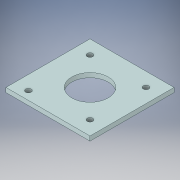
# Autodesk Inventor part: BASE_SOST.MEDIO
Saved by Autodesk Inventor 2019 (Build 230136000, 136)
## iProperties
Created: 2020-02-12
Part Number: BASE_SOST.MEDIO
Material: Genérico
Document SubType Name: Modeling
Designer: omar-
Density: 1 g/cm^3
Appearance: Valor por defecto
Author: omar-
Autodesk Inventor part; units mm, degrees
ref_plane "YZ Plane" through (0, 0, 0) normal (1, 0, 0) x (0, 1, 0)
ref_plane "XZ Plane" through (0, 0, 0) normal (0, 1, 0) x (-1, 0, 0)
ref_plane "XY Plane" through (0, 0, 0) normal (0, 0, 1) x (1, 0, 0)
sketch "Boceto1" plane through (0, 0, 0) normal (0, 1, 0) x (-1, 0, 0)
  circle A0 centre (0, 0) radius 13
  line L0 (-30, 30) -> (30, 30)
  line L1 (30, 30) -> (30, -30)
  line L2 (30, -30) -> (-30, -30)
  line L3 (-30, -30) -> (-30, 30)
  line L4 (-30, 30) -> (30, -30) construction
  line L5 (30, 30) -> (-30, -30) construction
  circle A1 centre (20, 24) radius 2
  circle A2 centre (20, -20) radius 2
  circle A3 centre (-20, -20) radius 2
  circle A4 centre (-20, 20) radius 2
  point P0 (0, 0)
  point P1 (0, 0)
  dimension "d0" = 26
  dimension "d1" = 60
  dimension "d2" = 60
  dimension "d3" = 4
  dimension "d4" = 4
  dimension "d5" = 4
  dimension "d6" = 4
  dimension "d7" = 40
  dimension "d8" = 20
  dimension "d9" = 20
  dimension "d10" = 40
  dimension "d11" = 40
  dimension "d12" = 20
  dimension "d13" = 40
  dimension "d14" = 20
  constraints: 12 end point, 5 centre point, 3 midpoint, 2 coincident, 2 parallel, 1 horizontal, 1 perpendicular
  measures "d0" diameter of A0
  measures "d1" distance of L1.end L2.end
  measures "d2" distance of L0.end L1.end
  measures "d3" diameter of A1
  measures "d4" diameter of A2
  measures "d5" diameter of A3
  measures "d6" diameter of A4
  measures "d8" horizontal distance of A2.centre point (0, 0)
  measures "d9" horizontal distance of point (0, 0) A1.centre
  measures "d10" horizontal distance of A4.centre A1.centre
  measures "d11" distance of A3.centre A4.centre
  measures "d12" horizontal distance of point (0, 0) A2.centre
  measures "d13" distance of A2.centre A3.centre
  measures "d14" horizontal distance of point (0, 0) A3.centre
extrude "Extrusión1" add sketch "Boceto1" along normal blind 3.18
